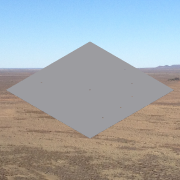
# Autodesk Inventor part: 0fasteners
Saved by Autodesk Inventor 2014 SP1 (Build 180222100, 222)
## iProperties
Created: 2013-12-02
Part Number: 0fasteners
Material: Generic
Document SubType Name: Modeling
Designer: David DeBoer
Density: 1 g/cm^3
Description: catch all for fasteners
Mass: 1.0151e+07 g
Surface Area: 8.01464e+06 cm^2
Volume: 1.0151e+07 cm^3
Appearance: Default
Author: Dave
Autodesk Inventor part; units mm, degrees
ref_plane "YZ Plane" through (0, 0, 0) normal (1, 0, 0) x (0, 1, 0)
ref_plane "XZ Plane" through (0, 0, 0) normal (0, 1, 0) x (-1, 0, 0)
ref_plane "XY Plane" through (0, 0, 0) normal (0, 0, 1) x (1, 0, 0)
sketch "Sketch1" plane through (0, 0, 0) normal (0, 1, 0) x (-1, 0, 0)
  line L0 (0, 0) -> (20000, 0)
  line L1 (20000, 0) -> (20000, 20000)
  line L2 (20000, 20000) -> (0, 20000)
  line L3 (0, 20000) -> (0, 0)
  dimension "d0" = 20000
  dimension "d1" = 20000
  constraints: 8 end point, 2 parallel, 1 horizontal, 1 perpendicular
  measures "d0" distance of L0.start L0.end
  measures "d1" distance of L2.end L0.start
extrude "Extrusion1" add sketch "Sketch1" along normal blind 25.4
sketch "Sketch2" plane through (0, 25.4, 0) normal (0, 1, 0) x (1, 0, 0)
  circle A0 centre (-10025, -10000) radius 127
  circle A1 centre (-10025, -1570) radius 127
  circle A2 centre (-2675, -10000) radius 127
  circle A3 centre (-17325.5942, -14215) radius 127
  circle A4 centre (-2724.4058, -14215) radius 127
  circle A5 centre (-3659.7133, -6325) radius 127
  circle A6 centre (-6350, -3634.7133) radius 127
  dimension "d4" = 254
  dimension "d5" = 254
  dimension "d6" = 8430
  dimension "d7" = 254
  dimension "d8" = 7350
  dimension "d11" = 360
  dimension "d15" = 60
  constraints: 7 centre point, 12 other
  measures "d4" diameter of A0
  measures "d5" diameter of A1
  measures "d6" distance of A0.centre A1.centre
  measures "d7" diameter of A2
  measures "d8" distance of A2.centre A0.centre
extrude "Extrusion2" cut sketch "Sketch2" against normal blind 25.4
body "Solid1"
